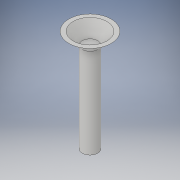
# Autodesk Inventor part: Part4
Saved by Autodesk Inventor 2018 (Build 220112000, 112)
## iProperties
Created: 2018-10-16
Part Number: Part4
Material: Generic
Document SubType Name: Modeling
Designer: Abhay
Density: 1 g/cm^3
Appearance: Default
Author: Abhay
Autodesk Inventor part; units mm, degrees
ref_plane "YZ Plane" through (0, 0, 0) normal (1, 0, 0) x (0, 1, 0)
ref_plane "XZ Plane" through (0, 0, 0) normal (0, 1, 0) x (-1, 0, 0)
ref_plane "XY Plane" through (0, 0, 0) normal (0, 0, 1) x (1, 0, 0)
sketch "Sketch1" plane through (0, 0, 0) normal (0, 0, 1) x (1, 0, 0)
  line L0 (0, 0) -> (20, 0)
  line L1 (20, 0) -> (7.2812, -11.3621)
  line L2 (7.2812, -11.3621) -> (7.2812, -96.3621)
  line L3 (7.2812, -96.3621) -> (0, -96.3621)
  line L4 (0, -96.3621) -> (0, 0)
  dimension "d0" = 20
  dimension "d1" = 85
  constraints: 10 end point, 3 perpendicular, 1 horizontal
  measures "d0" distance of L0.start L0.end
  measures "d1" distance of L1.end L2.end
revolve "Revolution1" add sketch "Sketch1" angle 360 about axis through (0, -96.3621, 0) along (0, 1, 0)
sketch "Sketch2" plane through (0, 0, 0) normal (0, 1, 0) x (1, 0, 0)
  circle A0 centre (0, 0) radius 16
  dimension "d3" = 32
  constraints: 1 centre point, 1 coincident
  measures "d3" diameter of A0
loft "Loft1" cut profiles "Sketch2" section 2 edges at (-7.2812, -11.3621, 0)
body "Solid1"
